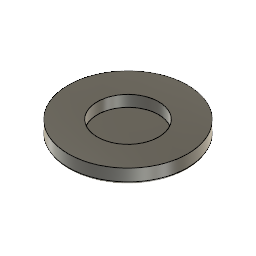
Spool Cover v3 (Autodesk Fusion 360 design; units mm, degrees)
Autodesk Fusion 360 part; units mm, degrees
cylinder "CylinderPrimitive1" add diameter 40 height 5 placed x (1, 0, 0) y (0, 1, 0) z (0, 0, 1) at (0, 0, 0)
hole "Hole1" at (0, 0, 5) direction (0, 0, -1) diameter 20.5 depth 3.75 tip angle 180
fillet "Fillet1" radius 1 1 edges at (-18.6465, 7.2323, 0)
